Autodesk Inventor part; units mm, degrees
(part 2 of 2)
sketch "スケッチ12" plane through (250, 25, -10) normal (0, 0, -1) x (-1, 0, 0)
  line L0 (248, -6.708245) -> (248, -43.291755)
  line L1 (248, -43.291755) -> (227.966174, -25)
  line L2 (227.966174, -25) -> (248, -6.708245)
  line L3 (252, -43.291755) -> (252, -6.708245)
  line L4 (252, -6.708245) -> (272.033826, -25)
  line L5 (272.033826, -25) -> (252, -43.291755)
  line L6 (452, -45.171573) -> (452, -6.764892)
  line L7 (452, -6.764892) -> (471.64993, -25.521643)
  line L8 (471.64993, -25.521643) -> (452, -45.171573)
  line L9 (404.966174, -46) -> (425, -27.708245)
  line L10 (425, -27.708245) -> (445.033826, -46)
  line L11 (445.033826, -46) -> (404.966174, -46)
  line L12 (372.033826, -25) -> (352, -43.291755)
  line L13 (352, -43.291755) -> (352, -6.708245)
  line L14 (352, -6.708245) -> (372.033826, -25)
  line L15 (322.033826, -25) -> (302, -43.291755)
  line L16 (302, -43.291755) -> (302, -6.708245)
  line L17 (302, -6.708245) -> (322.033826, -25)
  line L18 (222.033826, -25) -> (202, -43.291755)
  line L19 (202, -43.291755) -> (202, -6.708245)
  line L20 (202, -6.708245) -> (222.033826, -25)
  line L21 (175, -27.708245) -> (195.033826, -46)
  line L22 (195.033826, -46) -> (154.966174, -46)
  line L23 (154.966174, -46) -> (175, -27.708245)
  line L24 (77.966174, -25) -> (98, -6.708245)
  line L25 (98, -6.708245) -> (98, -43.291755)
  line L26 (98, -43.291755) -> (77.966174, -25)
  line L27 (75, -27.708245) -> (95.033826, -46)
  line L28 (95.033826, -46) -> (54.966174, -46)
  line L29 (54.966174, -46) -> (75, -27.708245)
  line L30 (22.626674, -25.455101) -> (4, -43.235108)
  line L31 (4, -43.235108) -> (4, -6.828427)
  line L32 (4, -6.828427) -> (22.626674, -25.455101)
  line L33 (25.520878, -22.692451) -> (6.828427, -4)
  line L34 (6.828427, -4) -> (45.103446, -4)
  line L35 (45.103446, -4) -> (25.520878, -22.692451)
  line L36 (75, -22.291755) -> (54.966174, -4)
  line L37 (54.966174, -4) -> (95.033826, -4)
  line L38 (95.033826, -4) -> (75, -22.291755)
  line L39 (122.033826, -25) -> (102, -43.291755)
  line L40 (102, -43.291755) -> (102, -6.708245)
  line L41 (102, -6.708245) -> (122.033826, -25)
  line L42 (175, -22.291755) -> (154.966174, -4)
  line L43 (154.966174, -4) -> (195.033826, -4)
  line L44 (195.033826, -4) -> (175, -22.291755)
  line L45 (225, -22.291755) -> (204.966174, -4)
  line L46 (204.966174, -4) -> (245.033826, -4)
  line L47 (245.033826, -4) -> (225, -22.291755)
  line L48 (275, -22.291755) -> (254.966174, -4)
  line L49 (254.966174, -4) -> (295.033826, -4)
  line L50 (295.033826, -4) -> (275, -22.291755)
  line L51 (325, -22.291755) -> (304.966174, -4)
  line L52 (304.966174, -4) -> (345.033826, -4)
  line L53 (345.033826, -4) -> (325, -22.291755)
  line L54 (375, -22.291755) -> (354.966174, -4)
  line L55 (354.966174, -4) -> (395.033826, -4)
  line L56 (395.033826, -4) -> (375, -22.291755)
  line L57 (445.033826, -4) -> (425, -22.291755)
  line L58 (425, -22.291755) -> (404.966174, -4)
  line L59 (404.966174, -4) -> (445.033826, -4)
  line L60 (496, -6.828427) -> (496, -43.235108)
  line L61 (496, -43.235108) -> (477.373326, -25.455101)
  line L62 (477.373326, -25.455101) -> (496, -6.828427)
  line L63 (456.828427, -46) -> (474.544134, -28.284293)
  line L64 (474.544134, -28.284293) -> (493.103446, -46)
  line L65 (493.103446, -46) -> (456.828427, -46)
  line L66 (402, -43.291755) -> (402, -6.708245)
  line L67 (402, -6.708245) -> (422.033826, -25)
  line L68 (422.033826, -25) -> (402, -43.291755)
  line L69 (375, -27.708245) -> (395.033826, -46)
  line L70 (395.033826, -46) -> (354.966174, -46)
  line L71 (354.966174, -46) -> (375, -27.708245)
  line L72 (325, -27.708245) -> (345.033826, -46)
  line L73 (345.033826, -46) -> (304.966174, -46)
  line L74 (304.966174, -46) -> (325, -27.708245)
  line L75 (275, -27.708245) -> (295.033826, -46)
  line L76 (295.033826, -46) -> (254.966174, -46)
  line L77 (254.966174, -46) -> (275, -27.708245)
  line L78 (225, -27.708245) -> (245.033826, -46)
  line L79 (245.033826, -46) -> (204.966174, -46)
  line L80 (204.966174, -46) -> (225, -27.708245)
  line L81 (172.033826, -25) -> (152, -43.291755)
  line L82 (152, -43.291755) -> (152, -6.708245)
  line L83 (152, -6.708245) -> (172.033826, -25)
  line L84 (125, -22.291755) -> (104.966174, -4)
  line L85 (104.966174, -4) -> (145.033826, -4)
  line L86 (145.033826, -4) -> (125, -22.291755)
  line L87 (72.033826, -25) -> (52, -43.291755)
  line L88 (52, -43.291755) -> (52, -6.708245)
  line L89 (52, -6.708245) -> (72.033826, -25)
  line L90 (25.455866, -28.284293) -> (43.171573, -46)
  line L91 (43.171573, -46) -> (6.896554, -46)
  line L92 (6.896554, -46) -> (25.455866, -28.284293)
  line L93 (28.35007, -25.521643) -> (48, -6.764892)
  line L94 (48, -6.764892) -> (48, -45.171573)
  line L95 (48, -45.171573) -> (28.35007, -25.521643)
  line L96 (125, -27.708245) -> (145.033826, -46)
  line L97 (145.033826, -46) -> (104.966174, -46)
  line L98 (104.966174, -46) -> (125, -27.708245)
  line L99 (127.966174, -25) -> (148, -6.708245)
  line L100 (148, -6.708245) -> (148, -43.291755)
  line L101 (148, -43.291755) -> (127.966174, -25)
  line L102 (177.966174, -25) -> (198, -6.708245)
  line L103 (198, -6.708245) -> (198, -43.291755)
  line L104 (198, -43.291755) -> (177.966174, -25)
  line L105 (277.966174, -25) -> (298, -6.708245)
  line L106 (298, -6.708245) -> (298, -43.291755)
  line L107 (298, -43.291755) -> (277.966174, -25)
  line L108 (327.966174, -25) -> (348, -6.708245)
  line L109 (348, -6.708245) -> (348, -43.291755)
  line L110 (348, -43.291755) -> (327.966174, -25)
  line L111 (377.966174, -25) -> (398, -6.708245)
  line L112 (398, -6.708245) -> (398, -43.291755)
  line L113 (398, -43.291755) -> (377.966174, -25)
  line L114 (448, -6.708245) -> (448, -43.291755)
  line L115 (448, -43.291755) -> (427.966174, -25)
  line L116 (427.966174, -25) -> (448, -6.708245)
  line L117 (493.171573, -4) -> (474.479122, -22.692451)
  line L118 (474.479122, -22.692451) -> (454.896554, -4)
  line L119 (454.896554, -4) -> (493.171573, -4)
  line L120 (500, 0) -> (0, 0)
  line L121 (0, -50) -> (0, 0)
  line L122 (500, -50) -> (0, -50)
  line L123 (500, 0) -> (500, -50)
  point P0 (250, -25)
sketch "スケッチ12 outline for 押し出し19" plane through (250, 25, -10) normal (0, 0, -1) x (-1, 0, 0)
  line L0 (404.966174, -46) -> (445.033826, -46)
  line L1 (425, -27.708245) -> (404.966174, -46)
  line L2 (445.033826, -46) -> (425, -27.708245)
  line L3 (448, -6.708245) -> (427.966174, -25)
  line L4 (448, -43.291755) -> (448, -6.708245)
  line L5 (427.966174, -25) -> (448, -43.291755)
  line L6 (445.033826, -4) -> (404.966174, -4)
  line L7 (425, -22.291755) -> (445.033826, -4)
  line L8 (404.966174, -4) -> (425, -22.291755)
  line L9 (402, -43.291755) -> (422.033826, -25)
  line L10 (402, -6.708245) -> (402, -43.291755)
  line L11 (422.033826, -25) -> (402, -6.708245)
  line L12 (375, -27.708245) -> (354.966174, -46)
  line L13 (395.033826, -46) -> (375, -27.708245)
  line L14 (354.966174, -46) -> (395.033826, -46)
  line L15 (377.966174, -25) -> (398, -43.291755)
  line L16 (398, -6.708245) -> (377.966174, -25)
  line L17 (398, -43.291755) -> (398, -6.708245)
  line L18 (375, -22.291755) -> (395.033826, -4)
  line L19 (354.966174, -4) -> (375, -22.291755)
  line L20 (395.033826, -4) -> (354.966174, -4)
  line L21 (372.033826, -25) -> (352, -6.708245)
  line L22 (352, -43.291755) -> (372.033826, -25)
  line L23 (352, -6.708245) -> (352, -43.291755)
  line L24 (325, -27.708245) -> (304.966174, -46)
  line L25 (345.033826, -46) -> (325, -27.708245)
  line L26 (304.966174, -46) -> (345.033826, -46)
  line L27 (327.966174, -25) -> (348, -43.291755)
  line L28 (348, -6.708245) -> (327.966174, -25)
  line L29 (348, -43.291755) -> (348, -6.708245)
  line L30 (325, -22.291755) -> (345.033826, -4)
  line L31 (304.966174, -4) -> (325, -22.291755)
  line L32 (345.033826, -4) -> (304.966174, -4)
  line L33 (322.033826, -25) -> (302, -6.708245)
  line L34 (302, -43.291755) -> (322.033826, -25)
  line L35 (302, -6.708245) -> (302, -43.291755)
  line L36 (275, -27.708245) -> (254.966174, -46)
  line L37 (295.033826, -46) -> (275, -27.708245)
  line L38 (254.966174, -46) -> (295.033826, -46)
  line L39 (277.966174, -25) -> (298, -43.291755)
  line L40 (298, -6.708245) -> (277.966174, -25)
  line L41 (298, -43.291755) -> (298, -6.708245)
  line L42 (275, -22.291755) -> (295.033826, -4)
  line L43 (254.966174, -4) -> (275, -22.291755)
  line L44 (295.033826, -4) -> (254.966174, -4)
  line L45 (252, -43.291755) -> (272.033826, -25)
  line L46 (252, -6.708245) -> (252, -43.291755)
  line L47 (272.033826, -25) -> (252, -6.708245)
  line L48 (225, -27.708245) -> (204.966174, -46)
  line L49 (245.033826, -46) -> (225, -27.708245)
  line L50 (204.966174, -46) -> (245.033826, -46)
  line L51 (248, -6.708245) -> (227.966174, -25)
  line L52 (248, -43.291755) -> (248, -6.708245)
  line L53 (227.966174, -25) -> (248, -43.291755)
  line L54 (225, -22.291755) -> (245.033826, -4)
  line L55 (204.966174, -4) -> (225, -22.291755)
  line L56 (245.033826, -4) -> (204.966174, -4)
  line L57 (222.033826, -25) -> (202, -6.708245)
  line L58 (202, -43.291755) -> (222.033826, -25)
  line L59 (202, -6.708245) -> (202, -43.291755)
  line L60 (175, -27.708245) -> (154.966174, -46)
  line L61 (195.033826, -46) -> (175, -27.708245)
  line L62 (154.966174, -46) -> (195.033826, -46)
  line L63 (177.966174, -25) -> (198, -43.291755)
  line L64 (198, -6.708245) -> (177.966174, -25)
  line L65 (198, -43.291755) -> (198, -6.708245)
  line L66 (175, -22.291755) -> (195.033826, -4)
  line L67 (154.966174, -4) -> (175, -22.291755)
  line L68 (195.033826, -4) -> (154.966174, -4)
  line L69 (172.033826, -25) -> (152, -6.708245)
  line L70 (152, -43.291755) -> (172.033826, -25)
  line L71 (152, -6.708245) -> (152, -43.291755)
  line L72 (122.033826, -25) -> (102, -6.708245)
  line L73 (102, -43.291755) -> (122.033826, -25)
  line L74 (102, -6.708245) -> (102, -43.291755)
  line L75 (125, -27.708245) -> (104.966174, -46)
  line L76 (145.033826, -46) -> (125, -27.708245)
  line L77 (104.966174, -46) -> (145.033826, -46)
  line L78 (127.966174, -25) -> (148, -43.291755)
  line L79 (148, -6.708245) -> (127.966174, -25)
  line L80 (148, -43.291755) -> (148, -6.708245)
  line L81 (125, -22.291755) -> (145.033826, -4)
  line L82 (104.966174, -4) -> (125, -22.291755)
  line L83 (145.033826, -4) -> (104.966174, -4)
  line L84 (75, -27.708245) -> (54.966174, -46)
  line L85 (95.033826, -46) -> (75, -27.708245)
  line L86 (54.966174, -46) -> (95.033826, -46)
  line L87 (77.966174, -25) -> (98, -43.291755)
  line L88 (98, -6.708245) -> (77.966174, -25)
  line L89 (98, -43.291755) -> (98, -6.708245)
  line L90 (75, -22.291755) -> (95.033826, -4)
  line L91 (54.966174, -4) -> (75, -22.291755)
  line L92 (95.033826, -4) -> (54.966174, -4)
  line L93 (72.033826, -25) -> (52, -6.708245)
  line L94 (52, -43.291755) -> (72.033826, -25)
  line L95 (52, -6.708245) -> (52, -43.291755)
extrude "押し出し19" cut sketch "スケッチ12 outline for 押し出し19" against normal through all
